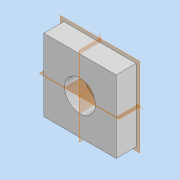
# Autodesk Inventor part: bearing1b
Saved by Autodesk Inventor 2022 (Build 260153000, 153)
## iProperties
Created: 2024-01-11
Part Number: bearing1b
Material: 一般
Document SubType Name: Modeling
Designer: ktamu
Density: 1 g/cm^3
Appearance: 既定
Author: ktamu
Autodesk Inventor part; units mm, degrees
sketch "スケッチ1" plane through (0, 0, 0) normal (0, 0, 1) x (1, 0, 0)
  circle A0 centre (0, 0) radius 10
  line L0 (-23.5, 23.5) -> (23.5, 23.5)
  line L1 (23.5, 23.5) -> (23.5, -23.5)
  line L2 (23.5, -23.5) -> (-23.5, -23.5)
  line L3 (-23.5, -23.5) -> (-23.5, 23.5)
  line L4 (-23.5, 23.5) -> (23.5, -23.5) construction
  line L5 (23.5, 23.5) -> (-23.5, -23.5) construction
  dimension "d0" = 20
  dimension "d1" = 47
  dimension "d2" = 47
  constraints: 12 end point, 2 midpoint, 2 parallel, 1 centre point, 1 coincident, 1 horizontal, 1 perpendicular
  measures "d0" diameter of A0
  measures "d1" distance of L1.end L2.end
  measures "d2" distance of L0.end L1.end
extrude "押し出し1" add sketch "スケッチ1" along normal blind 13
